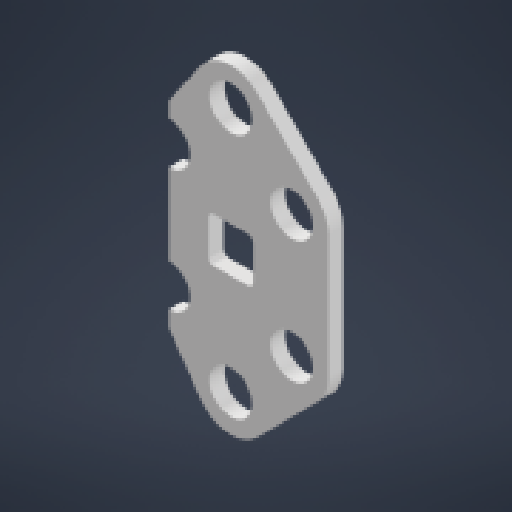
# Autodesk Inventor part: pto-shaft-support
Saved by Autodesk Inventor 2023.2 (Build 272271000, 271)
## iProperties
Created: 2023-03-20
Part Number: pto-shaft-support
Material: Generic
Document SubType Name: Modeling
Designer: Liam
Density: 1 g/cm^3
Appearance: Default
Author: Liam
Autodesk Inventor part; units mm, degrees
ref_plane "YZ Plane" through (0, 0, 0) normal (1, 0, 0) x (0, 1, 0)
ref_plane "XZ Plane" through (0, 0, 0) normal (0, 1, 0) x (-1, 0, 0)
ref_plane "XY Plane" through (0, 0, 0) normal (0, 0, 1) x (1, 0, 0)
sketch "Sketch1" plane through (0, 0, 0) normal (0, 0, 1) x (1, 0, 0)
  line L0 (0, 0) -> (0, -2.3114)
  line L1 (0, 0) -> (0, 2.3114)
  line L2 (0, 0) -> (2.3114, 0)
  line L3 (0, 0) -> (-2.3114, 0)
  line L4 (0, -2.3114) -> (-1.8034, -2.3114)
  line L5 (-2.3114, -1.8034) -> (-2.3114, 1.8034)
  line L6 (-1.8034, 2.3114) -> (1.8034, 2.3114)
  line L7 (2.3114, 1.8034) -> (2.3114, -1.8034)
  line L8 (1.8034, -2.3114) -> (0, -2.3114)
  arc A0 (1.8034, -2.3114) -> (2.3114, -1.8034) centre (1.8034, -1.8034) ccw
  arc A1 (-2.3114, -1.8034) -> (-1.8034, -2.3114) centre (-1.8034, -1.8034) ccw
  arc A2 (-1.8034, 2.3114) -> (-2.3114, 1.8034) centre (-1.8034, 1.8034) ccw
  arc A3 (2.3114, 1.8034) -> (1.8034, 2.3114) centre (1.8034, 1.8034) ccw
  circle A4 centre (6.2738, -6.35) radius 2.1844 projected
  circle A5 centre (6.2738, 6.35) radius 2.1844 projected
  line L9 (-6.4262, -10.16) -> (-6.4262, -8.5344)
  line L10 (-6.4262, -2.54) -> (-6.4262, -4.1656)
  arc A6 (-6.4262, -8.5344) -> (-6.4262, -4.1656) centre (-6.4262, -6.35) ccw
  arc A7 (-6.4262, 4.1656) -> (-6.4262, 8.5344) centre (-6.4262, 6.35) ccw
  line L11 (-6.4262, 2.54) -> (-6.4262, 4.1656)
  line L12 (-6.4262, 8.5344) -> (-6.4262, 10.16)
  circle A8 centre (0, -12.7) radius 2.1971 projected
  circle A9 centre (0, 12.7) radius 2.1971 projected
  line L13 (-3.122, 14.8838) -> (-6.4262, 10.16)
  line L14 (-6.4262, -10.16) -> (-3.122, -14.8838)
  line L15 (8.9841, -9.0278) -> (2.7103, -15.3778)
  line L16 (10.0838, -6.35) -> (10.0838, 6.35)
  line L17 (8.9841, 9.0278) -> (2.7103, 15.3778)
  arc A10 (-3.122, -14.8838) -> (2.7103, -15.3778) centre (0, -12.7) ccw
  arc A11 (8.9841, -9.0278) -> (10.0838, -6.35) centre (6.2738, -6.35) ccw
  arc A12 (10.0838, 6.35) -> (8.9841, 9.0278) centre (6.2738, 6.35) ccw
  arc A13 (2.7103, 15.3778) -> (-3.122, 14.8838) centre (0, 12.7) ccw
  line L18 (-6.4262, 2.54) -> (-6.4262, -2.54)
  point P0 (2.3114, -2.3114)
  dimension "d0" = 2.3114
  dimension "d1" = 2.3114
  dimension "d2" = 2.3114
  dimension "d3" = 2.3114
  dimension "d4" = 0.508
  constraints: 38 end point, 20 point on circle, 10 centre point, 8 tangent, 7 vertical, 5 horizontal, 4 perpendicular, 4 point on line, 3 equal radius, 8 other
  measures "d0" distance of L0.start L0.end
  measures "d1" distance of L0.start L1.end
  measures "d2" distance of L0.start L2.end
  measures "d3" distance of L0.start L3.end
  measures "d4" radius of A0
extrude "Extrusion1" add sketch "Sketch1" along normal blind 1.524
body "Solid1"
